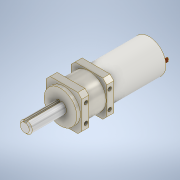
# Autodesk Inventor part: rs550_p60s-4-57
Saved by Autodesk Inventor 2020.2 (Build 242310000, 310)
## iProperties
Created: 2019-11-09
Part Number: rs550_p60s-4-57
Material: Titanium
Document SubType Name: Modeling
Designer: agmle
Density: 4.51 g/cm^3
Appearance: Titanium
Mass: 475.407 g
Surface Area: 175.135 cm^2
Volume: 105.412 cm^3
Author: agmle
Autodesk Inventor part; units mm, degrees
ref_plane "YZ Plane" through (0, 0, 0) normal (1, 0, 0) x (0, 1, 0)
ref_plane "XZ Plane" through (0, 0, 0) normal (0, 1, 0) x (-1, 0, 0)
ref_plane "XY Plane" through (0, 0, 0) normal (0, 0, 1) x (1, 0, 0)
sketch "Sketch1" plane through (0, 0, 0) normal (0, 0, 1) x (1, 0, 0)
  line L0 (-19.05, 19.05) -> (19.05, 19.05)
  line L1 (19.05, 19.05) -> (19.05, -19.05)
  line L2 (19.05, -19.05) -> (-19.05, -19.05)
  line L3 (-19.05, -19.05) -> (-19.05, 19.05)
  line L4 (0, 19.05) -> (0, -19.05) construction
  point P0 (0, 0)
  point P1 (0, 0)
  dimension "d0" = 38.1
  dimension "d1" = 38.1
  constraints: 10 end point, 3 midpoint, 2 parallel, 1 coincident, 1 horizontal, 1 perpendicular
  measures "d0" distance of L2.end L0.start
  measures "d1" distance of L0.start L0.end
extrude "Extrusion1" add sketch "Sketch1" along normal blind 7.5692
sketch "Sketch2" plane through (0, 0, 7.5692) normal (0, 0, 1) x (1, 0, 0)
  circle A0 centre (0, 0) radius 17.5006
  dimension "d4" = 35.0012
  constraints: 1 centre point, 1 coincident
  measures "d4" diameter of A0
extrude "Extrusion2" add sketch "Sketch2" along normal blind 3.7338
sketch "Sketch3" plane through (0, 0, 11.303) normal (0, 0, 1) x (1, 0, 0)
  arc A0 (-1.524, 6.1644) -> (1.524, 6.1644) centre (0, 0) ccw
  line L0 (-1.524, 4.5769) -> (1.524, 4.5769)
  line L1 (1.524, 4.5769) -> (1.524, 6.1644)
  line L2 (-1.524, 4.5769) -> (-1.524, 6.1644)
  dimension "d7" = 12.7
  dimension "d8" = 3.048
  dimension "d9" = 1.5875
  constraints: 6 end point, 2 parallel, 2 point on circle, 1 centre point, 1 coincident, 1 horizontal, 1 perpendicular
  measures "d7" diameter of A0
  measures "d8" distance of L0.start L0.end
  measures "d9" distance of L0.start L2.end
extrude "Extrusion3" add sketch "Sketch3" along normal blind 38.1
sketch "Sketch4" plane through (0, 0, 0) normal (0, 0, -1) x (-1, 0, 0)
  circle A0 centre (0, 0) radius 18.415
  dimension "d12" = 36.83
  constraints: 1 centre point, 1 coincident
  measures "d12" diameter of A0
extrude "Extrusion4" add sketch "Sketch4" along normal blind 19.05
sketch "Sketch5" plane through (0, 0, -19.05) normal (0, 0, -1) x (-1, 0, 0)
  line L0 (-19.05, 19.05) -> (19.05, 19.05) projected
  line L1 (-19.05, -19.05) -> (-19.05, 19.05) projected
  line L2 (19.05, -19.05) -> (-19.05, -19.05) projected
  line L3 (19.05, 19.05) -> (19.05, -19.05) projected
  point P0 (0, 0)
extrude "Extrusion5" add sketch "Sketch5" along normal blind 7.62
sketch "Sketch6" plane through (0, 0, -26.67) normal (0, 0, -1) x (-1, 0, 0)
  circle A0 centre (0, 0) radius 17.78
  dimension "d17" = 35.56
  constraints: 1 centre point, 1 coincident
  measures "d17" diameter of A0
extrude "Extrusion6" add sketch "Sketch6" along normal blind 56.896
sketch "Sketch7" plane through (0, 0, -83.566) normal (0, 0, -1) x (-1, 0, 0)
  line L0 (-13.716, 1.905) -> (-12.7, 1.905)
  line L1 (-12.7, 1.905) -> (-12.7, -1.905)
  line L2 (-12.7, -1.905) -> (-13.716, -1.905)
  line L3 (-13.716, -1.905) -> (-13.716, 1.905)
  line L4 (12.7, 1.905) -> (13.716, 1.905)
  line L5 (13.716, 1.905) -> (13.716, -1.905)
  line L6 (13.716, -1.905) -> (12.7, -1.905)
  line L7 (12.7, -1.905) -> (12.7, 1.905)
  line L8 (-12.7, 0) -> (12.7, 0) construction
  point P0 (0, 0)
  point P1 (0, 0)
  dimension "d20" = 25.4
  dimension "d21" = 1.016
  dimension "d22" = 3.81
  constraints: 18 end point, 4 parallel, 3 midpoint, 2 horizontal, 2 perpendicular, 2 point on line, 1 coincident, 1 collinear
  measures "d20" distance between parallel lines of L7 L1
  measures "d21" distance of L5.end L6.end
  measures "d22" distance of L4.end L5.end
extrude "Extrusion7" add sketch "Sketch7" along normal blind 6.35
chamfer "Chamfer1" distance 4.191 angle 45 8 edges at (19.05, 19.05, 3.7846) (19.05, 19.05, -22.86) (19.05, -19.05, -22.86) (19.05, -19.05, 3.7846) (-19.05, -19.05, 3.7846) (-19.05, -19.05, -22.86) (-19.05, 19.05, -22.86) (-19.05, 19.05, 3.7846)
chamfer "Chamfer2" distance 1.5875 angle 45 1 edges at (0, -6.35, 49.403)
sketch "Sketch8" plane through (19.05, -14.859, -19.05) normal (1, 0, 0) x (0, 0, -1)
  line L0 (3.175, 24.384) -> (-22.225, 24.384) construction
  line L1 (-22.225, 24.384) -> (-22.225, 5.334) construction
  line L2 (-22.225, 5.334) -> (3.175, 5.334) construction
  line L3 (3.175, 5.334) -> (3.175, 24.384) construction
  line L4 (-9.525, 24.384) -> (-9.525, 5.334) construction
  line L5 (0, 0) -> (0, 29.718) construction
  line L6 (0, 14.859) -> (-19.05, 14.859) construction
  line L7 (-30.353, 32.3596) -> (-30.353, -2.6416) projected
  point P0 (-9.525, 14.859)
  dimension "d31" = 25.4
  dimension "d32" = 19.05
  dimension "d47" = 8.128
  constraints: 12 end point, 5 midpoint, 2 coincident, 2 horizontal, 2 parallel, 1 perpendicular
  measures "d31" distance of L0.start L0.end
  measures "d32" distance of L2.end L0.start
  measures "d47" distance between parallel lines of L7 L1
hole "Hole1" at (19.05, 9.525, -22.225) at (19.05, -9.525, -22.225) at (19.05, -9.525, 3.175) at (19.05, 9.525, 3.175) direction (-1, 0, 0) diameter 3.9624 depth 11.0744 tip angle 118 thread size "10-32 UNF" class "2B" standard "ANSI Unified Screw Threads"
sketch "Sketch9" plane through (-19.05, -14.859, -19.05) normal (-1, 0, 0) x (0, 0, 1)
  circle A0 centre (-3.175, 24.384) radius 1.9812 construction
  circle A1 centre (-3.175, 5.334) radius 1.9812 construction
  circle A2 centre (22.225, 5.334) radius 1.9812 construction
  circle A3 centre (22.225, 24.384) radius 1.9812 construction
  point P0 (19.05, 14.859)
  constraints: 4 coincident
hole "Hole2" at (-19.05, -9.525, -22.225) at (-19.05, 9.525, -22.225) at (-19.05, 9.525, 3.175) at (-19.05, -9.525, 3.175) direction (1, 0, 0) diameter 3.9624 depth 11.0744 tip angle 118 thread size "10-32 UNF" class "2B" standard "ANSI Unified Screw Threads"
body "Solid1"
